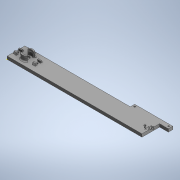
# Autodesk Inventor part: Arm Bottom Left
Saved by Autodesk Inventor 2020.5 (Build 245400000, 400)
## iProperties
Created: 2023-03-21
Part Number: Arm Bottom Left
Material: Generic
Document SubType Name: Modeling
Designer: Wes
Density: 1 g/cm^3
Appearance: Default
Author: Wes
Autodesk Inventor part; units mm, degrees
ref_plane "YZ Plane" through (0, 0, 0) normal (1, 0, 0) x (0, 1, 0)
ref_plane "XZ Plane" through (0, 0, 0) normal (0, 1, 0) x (-1, 0, 0)
ref_plane "XY Plane" through (0, 0, 0) normal (0, 0, 1) x (1, 0, 0)
sketch "Base" plane through (0, 0, 0) normal (0, 0, 1) x (1, 0, 0)
  line L0 (0, 0) -> (-30, 0)
  line L1 (-30, 0) -> (-30, 230)
  line L2 (-30, 230) -> (0, 230)
  line L3 (0, 230) -> (0, 0)
  dimension "d0" = 30
  dimension "d1" = 230
  constraints: 8 end point, 2 parallel, 1 horizontal, 1 perpendicular
  measures "d0" distance of L1.end L2.end
  measures "d1" distance of L0.end L1.end
sketch "Base outline for Extrusion1" plane through (0, 0, 0) normal (0, 0, 1) x (1, 0, 0)
  line L0 (0, 0) -> (0, 230)
  line L1 (-30, 0) -> (0, 0)
  line L2 (-30, 230) -> (-30, 0)
  line L3 (0, 230) -> (-30, 230)
extrude "Extrusion1" add sketch "Base outline for Extrusion1" along normal blind 5
sketch "Axle Screw Countersink" plane through (0, 0, 5) normal (0, 0, 1) x (1, 0, 0)
  line L0 (-15, 0) -> (-15, 20) construction
  circle A0 centre (-15, 20) radius 3.15
  dimension "d4" = 20
  dimension "d58" = 6.3
  constraints: 2 end point, 1 centre point, 1 coincident, 1 vertical
  measures "d4" distance of L0.start L0.end
  measures "d58" diameter of A0
sketch "Axle Screw Countersink outline for Extrusion2" plane through (0, 0, 5) normal (0, 0, 1) x (1, 0, 0)
  circle A0 centre (-15, 20) radius 3.15
extrude "Extrusion2" cut sketch "Axle Screw Countersink outline for Extrusion2" against normal blind 1.2
sketch "Motor Arm Center Fitting" plane through (0, 0, 5) normal (0, 0, 1) x (1, 0, 0)
  line L0 (-19.392963, 15.95) -> (-19.392963, 24.05) construction
  arc A0 (-19.392963, 24.05) -> (-19.392963, 15.95) centre (-15, 20) ccw
  line L1 (-19.392963, 15.95) -> (-21.231023, 14.255439)
  line L2 (-19.392963, 24.05) -> (-21.231023, 25.744561)
  line L3 (-15, 8.350441) -> (-15, 30.698869) construction
  arc A1 (-21.231023, 25.744561) -> (-21.231023, 14.255439) centre (-15, 20) ccw
  line L4 (-10.607037, 15.95) -> (-10.607037, 24.05) construction
  line L5 (-10.607037, 15.95) -> (-19.392963, 15.95) construction
  arc A2 (-10.607037, 15.95) -> (-10.607037, 24.05) centre (-15, 20) ccw
  line L6 (-10.607037, 15.95) -> (-8.768977, 14.255439)
  line L7 (-10.607037, 24.05) -> (-8.768977, 25.744561)
  arc A3 (-8.768977, 14.255439) -> (-8.768977, 25.744561) centre (-15, 20) ccw
  circle A4 centre (-15, 20) radius 5.975 construction
  point P0 (0, 0)
  point P1 (-15, 20)
  dimension "d18" = 11.95
  dimension "d19" = 8.1
  dimension "d20" = 8.1
  dimension "d21" = 2.5
  dimension "d22" = 2.5
  constraints: 16 end point, 12 point on circle, 5 centre point, 2 line through centre, 2 symmetric about line, 2 vertical, 1 concentric, 1 perpendicular, 2 other
  measures "d18" diameter of A4
  measures "d19" distance of L5.start L4.end
  measures "d20" distance of L5.end L0.end
  measures "d21" distance of L5.end L1.end
  measures "d22" distance of L0.end L2.end
sketch "Motor Arm Center Fitting outline for Extrusion3" plane through (0, 0, 5) normal (0, 0, 1) x (1, 0, 0)
  arc A0 (-10.607037, 24.05) -> (-10.607037, 15.95) centre (-15, 20) cw
  line L0 (-8.768977, 25.744561) -> (-10.607037, 24.05)
  arc A1 (-8.768977, 14.255439) -> (-8.768977, 25.744561) centre (-15, 20) ccw
  line L1 (-10.607037, 15.95) -> (-8.768977, 14.255439)
  arc A2 (-21.231023, 25.744561) -> (-21.231023, 14.255439) centre (-15, 20) ccw
  line L2 (-19.392963, 24.05) -> (-21.231023, 25.744561)
  arc A3 (-19.392963, 15.95) -> (-19.392963, 24.05) centre (-15, 20) cw
  line L3 (-21.231023, 14.255439) -> (-19.392963, 15.95)
extrude "Extrusion3" add sketch "Motor Arm Center Fitting outline for Extrusion3" along normal blind 5
sketch "Motor Rotation Support" plane through (0, 0, 10) normal (0, 0, 1) x (1, 0, 0)
  line L0 (-20.975, 20) -> (-21.775, 20) construction
  circle A0 centre (-15, 20) radius 6.775 construction
  arc A1 (-19.981142, 24.592259) -> (-19.981142, 15.407741) centre (-15, 20) ccw
  line L1 (-21.775, 20) -> (-23.775, 20) construction
  circle A2 centre (-15, 20) radius 8.775 construction
  arc A3 (-21.45159, 25.947908) -> (-21.45159, 14.052092) centre (-15, 20) ccw
  line L2 (-21.45159, 14.052092) -> (-19.981142, 15.407741)
  line L3 (-19.981142, 24.592259) -> (-21.45159, 25.947908)
  line L4 (-15, 8.529475) -> (-15, 32.047921) construction
  line L5 (-8.54841, 14.052092) -> (-10.018858, 15.407741)
  arc A4 (-8.54841, 14.052092) -> (-8.54841, 25.947908) centre (-15, 20) ccw
  arc A5 (-10.018858, 15.407741) -> (-10.018858, 24.592259) centre (-15, 20) ccw
  line L6 (-10.018858, 24.592259) -> (-8.54841, 25.947908)
  point P0 (0, 0)
  point P1 (-21.231023, 14.255439)
  point P2 (-21.231023, 25.744561)
  dimension "d25" = 0.8
  dimension "d26" = 2
  constraints: 16 point on circle, 14 end point, 6 centre point, 4 symmetric about line, 2 coincident, 2 horizontal, 1 concentric, 1 vertical, 2 other
  measures "d25" distance of L0.start L0.end
  measures "d26" distance of L0.end L1.end
sketch "Motor Rotation Support outline for Extrusion4" plane through (0, 0, 10) normal (0, 0, 1) x (1, 0, 0)
  arc A0 (-8.54841, 14.052092) -> (-8.54841, 25.947908) centre (-15, 20) ccw
  line L0 (-10.018858, 15.407741) -> (-8.54841, 14.052092)
  arc A1 (-10.018858, 24.592259) -> (-10.018858, 15.407741) centre (-15, 20) cw
  line L1 (-8.54841, 25.947908) -> (-10.018858, 24.592259)
  arc A2 (-21.45159, 25.947908) -> (-21.45159, 14.052092) centre (-15, 20) ccw
  line L2 (-19.981142, 24.592259) -> (-21.45159, 25.947908)
  arc A3 (-19.981142, 15.407741) -> (-19.981142, 24.592259) centre (-15, 20) cw
  line L3 (-21.45159, 14.052092) -> (-19.981142, 15.407741)
extrude "Extrusion4" add sketch "Motor Rotation Support outline for Extrusion4" along normal blind 3.35
sketch "Motor Arm Screw Holes" plane through (0, 0, 5) normal (0, 0, 1) x (1, 0, 0)
  line L0 (-15, 20) -> (-15, 37.1) construction
  line L1 (-15, 20) -> (-15, 2.9) construction
  line L2 (-15, 20) -> (-15, 4.2) construction
  line L3 (-15, 20) -> (-15, 35.8) construction
  line L4 (-15, 4.2) -> (-15, 2.9) construction
  line L5 (-15, 35.8) -> (-15, 37.1) construction
  circle A0 centre (-15, 36.45) radius 1.175
  circle A1 centre (-15, 3.55) radius 1.175
  point P0 (0, 0)
  dimension "d59" = 34.2
  dimension "d60" = 31.6
  dimension "d61" = 2.35
  dimension "d62" = 2.35
  constraints: 12 end point, 3 vertical, 2 centre point, 2 midpoint, 2 point on line, 1 coincident, 1 collinear
  measures "d59" distance of L0.end L1.end
  measures "d60" distance of L3.end L2.end
  measures "d61" diameter of A0
  measures "d62" diameter of A1
sketch "Motor Arm Screw Holes outline for Extrusion5" plane through (0, 0, 5) normal (0, 0, 1) x (1, 0, 0)
  circle A0 centre (-15, 36.45) radius 1.175
  circle A1 centre (-15, 3.55) radius 1.175
extrude "Extrusion5" cut sketch "Motor Arm Screw Holes outline for Extrusion5" against normal through all
sketch "Motor Arm Support" plane through (0, 0, 5) normal (0, 0, 1) x (1, 0, 0)
  line L0 (-15, 2.375) -> (-15, 6.875) construction
  line L1 (-15, 6.875) -> (-11.875, 6.875) construction
  line L2 (-15, 6.875) -> (-18.125, 6.875) construction
  line L3 (-21.064431, 20.215447) -> (-9.114431, 20.215447) construction
  line L4 (-15, 3.55) -> (-12.2, 3.55) construction
  line L5 (-15, 3.55) -> (-12.2, 3.55) construction
  line L6 (-15, 3.55) -> (-17.8, 3.55) construction
  line L7 (-15, 3.55) -> (-12.2, 3.55) construction
  line L8 (-18.125, 6.875) -> (-17.8, 3.55)
  line L9 (-17.8, 3.55) -> (-19.790514, 3.355438)
  line L10 (-19.790514, 3.355438) -> (-20.115514, 6.680438)
  line L11 (-20.115514, 6.680438) -> (-18.125, 6.875)
  line L12 (-11.875, 6.875) -> (-12.2, 3.55)
  line L13 (-12.2, 3.55) -> (-10.209486, 3.355438)
  line L14 (-9.884486, 6.680438) -> (-11.875, 6.875)
  line L15 (-10.209486, 3.355438) -> (-9.884486, 6.680438)
  line L16 (-17.8, 3.55) -> (-17.605438, 1.559486)
  line L17 (-17.605438, 1.559486) -> (-19.595952, 1.364925)
  line L18 (-19.595952, 1.364925) -> (-19.790514, 3.355438)
  line L19 (-12.2, 3.55) -> (-12.394562, 1.559486)
  line L20 (-12.394562, 1.559486) -> (-10.404048, 1.364925)
  line L21 (-10.404048, 1.364925) -> (-10.209486, 3.355438)
  line L22 (-17.8, 36.880894) -> (-19.790514, 37.075456)
  line L23 (-17.8, 36.880894) -> (-17.605438, 38.871408)
  line L24 (-17.605438, 38.871408) -> (-19.595952, 39.06597)
  line L25 (-19.595952, 39.06597) -> (-19.790514, 37.075456)
  line L26 (-18.125, 33.555894) -> (-17.8, 36.880894)
  line L27 (-19.790514, 37.075456) -> (-20.115514, 33.750456)
  line L28 (-20.115514, 33.750456) -> (-18.125, 33.555894)
  line L29 (-11.875, 33.555894) -> (-12.2, 36.880894)
  line L30 (-12.394562, 38.871408) -> (-10.404048, 39.06597)
  line L31 (-12.2, 36.880894) -> (-10.209486, 37.075456)
  line L32 (-10.404048, 39.06597) -> (-10.209486, 37.075456)
  line L33 (-10.209486, 37.075456) -> (-9.884486, 33.750456)
  line L34 (-9.884486, 33.750456) -> (-11.875, 33.555894)
  line L35 (-12.2, 36.880894) -> (-12.394562, 38.871408)
  point P0 (0, 0)
  dimension "d63" = 4.5
  dimension "d64" = 6.25
  dimension "d65" = 5.6
  dimension "d66" = 2
  dimension "d67" = 2
  constraints: 72 end point, 18 symmetric about line, 7 horizontal, 5 perpendicular, 2 collinear, 1 vertical
  measures "d63" distance of L0.start L1.start
  measures "d64" distance of L2.end L1.end
  measures "d65" distance of L8.end L4.end
  measures "d66" distance of L8.end L10.start
  measures "d67" distance of L8.end L17.start
sketch "Motor Arm Support outline for Extrusion6" plane through (0, 0, 5) normal (0, 0, 1) x (1, 0, 0)
  line L0 (-11.875, 6.875) -> (-12.394562, 1.559486)
  line L1 (-12.394562, 1.559486) -> (-10.404048, 1.364925)
  line L2 (-10.404048, 1.364925) -> (-9.884486, 6.680438)
  line L3 (-9.884486, 6.680438) -> (-11.875, 6.875)
  line L4 (-20.115514, 6.680438) -> (-19.595952, 1.364925)
  line L5 (-19.595952, 1.364925) -> (-17.605438, 1.559486)
  line L6 (-17.605438, 1.559486) -> (-18.125, 6.875)
  line L7 (-18.125, 6.875) -> (-20.115514, 6.680438)
  line L8 (-9.884486, 33.750456) -> (-10.404048, 39.06597)
  line L9 (-10.404048, 39.06597) -> (-12.394562, 38.871408)
  line L10 (-12.394562, 38.871408) -> (-11.875, 33.555894)
  line L11 (-11.875, 33.555894) -> (-9.884486, 33.750456)
  line L12 (-18.125, 33.555894) -> (-17.605438, 38.871408)
  line L13 (-17.605438, 38.871408) -> (-19.595952, 39.06597)
  line L14 (-19.595952, 39.06597) -> (-20.115514, 33.750456)
  line L15 (-20.115514, 33.750456) -> (-18.125, 33.555894)
extrude "Extrusion6" add sketch "Motor Arm Support outline for Extrusion6" along normal blind 3
draft "FaceDraft1" angle 28 pull direction (0, 0, 1) faces at (-10.23086, 3.136763, 6) (-10.057673, 35.522294, 6) fixed edges at (-10.144267, 4.022682, 8) (-10.144267, 36.408213, 8)
draft "FaceDraft2" angle 28 pull direction (0, 0, 1) faces at (-19.76914, 37.294132, 6) (-19.942327, 4.9086, 6) fixed edges at (-19.855733, 36.408213, 8) (-19.855733, 4.022682, 8)
fillet "Fillet1" radius 2 4 edges at (-23.475, 20, 5) (-6.525, 20, 5) (-8.225, 20, 10) (-21.775, 20, 10)
sketch "Axle Hole" plane through (0, 0, 5) normal (0, 0, 1) x (1, 0, 0)
  line L0 (0, 230) -> (-30, 230) construction
  line L1 (-15, 230) -> (-15, 220) construction
  circle A0 centre (-15, 220) radius 1.5
  point P0 (0, 0)
  dimension "d73" = 10
  dimension "d74" = 3
  constraints: 2 end point, 1 centre point, 1 coincident, 1 midpoint, 1 vertical
  measures "d73" distance of L1.start L1.end
  measures "d74" diameter of A0
sketch "Axle Hole outline for Extrusion7" plane through (0, 0, 5) normal (0, 0, 1) x (1, 0, 0)
  circle A0 centre (-15, 220) radius 1.5
extrude "Extrusion7" cut sketch "Axle Hole outline for Extrusion7" against normal through all
sketch "Motor Backplate Offset" plane through (0, 0, 0) normal (0, 0, -1) x (-1, 0, 0)
  circle A0 centre (15, 220) radius 1.5 construction
  line L0 (15, 220) -> (15, 180) construction
  line L1 (15, 220) -> (15, 240) construction
  line L2 (33.5, 240) -> (33.5, 180)
  line L3 (33.5, 180) -> (30, 180)
  line L4 (30, 180) -> (30, 240)
  line L5 (30, 240) -> (30, 245)
  line L6 (30, 245) -> (33.5, 245)
  line L7 (33.5, 245) -> (33.5, 240)
  line L8 (30, 230) -> (30, 245)
  point P0 (0, 0)
  dimension "d77" = 40
  dimension "d78" = 20
  dimension "d83" = 3.5
  dimension "d84" = 60
  dimension "d142" = 5
  constraints: 18 end point, 2 parallel, 2 vertical
  measures "d77" distance of L0.start L0.end
  measures "d78" distance of L0.start L1.end
  measures "d83" distance of L2.end L3.end
  measures "d84" distance of L0.end L1.end
  measures "d142" distance of L5.start L5.end
sketch "Motor Backplate Offset outline for Extrusion8" plane through (0, 0, 0) normal (0, 0, -1) x (-1, 0, 0)
  line L0 (30, 240) -> (30, 180)
  line L1 (30, 245) -> (30, 240)
  line L2 (33.5, 245) -> (30, 245)
  line L3 (33.5, 240) -> (33.5, 245)
  line L4 (33.5, 180) -> (33.5, 240)
  line L5 (30, 180) -> (33.5, 180)
extrude "Extrusion8" add sketch "Motor Backplate Offset outline for Extrusion8" against normal up to surface (5 mm away)
sketch "Reference" plane through (0, 0, 0) normal (0, 0, -1) x (-1, 0, 0)
  circle A0 centre (15, 220) radius 1.5 construction
  line L0 (15, 220) -> (24.935, 220) construction
  point P0 (0, 0)
  dimension "d98" = 9.935
  constraints: 2 end point, 1 horizontal
  measures "d98" distance of L0.start L0.end
sketch "Motor Backplate Offset 2" plane through (0, 0, 0) normal (0, 0, -1) x (-1, 0, 0)
  line L0 (33.5, 180) -> (33.5, 245) projected
  line L1 (33.5, 245) -> (37.5, 245)
  line L2 (37.5, 245) -> (37.5, 180)
  line L3 (37.5, 180) -> (33.5, 180)
  line L4 (33.5, 180) -> (33.5, 245)
  point P0 (0, 0)
  dimension "d144" = 4
  constraints: 8 end point, 2 parallel, 1 horizontal, 1 perpendicular
  measures "d144" distance of L2.end L3.end
sketch "Motor Backplate Offset 2 outline for Extrusion17" plane through (0, 0, 0) normal (0, 0, -1) x (-1, 0, 0)
  line L0 (33.5, 180) -> (37.5, 180)
  line L1 (33.5, 245) -> (33.5, 180)
  line L2 (37.5, 245) -> (33.5, 245)
  line L3 (37.5, 180) -> (37.5, 245)
extrude "Extrusion17" add sketch "Motor Backplate Offset 2 outline for Extrusion17" against normal up to surface (5 mm away)
sketch "Connector Screw Holes" plane through (0, 0, 0) normal (0, 0, -1) x (-1, 0, 0)
  line L0 (37.5, 180) -> (37.5, 245) construction
  line L1 (37.5, 245) -> (37.5, 241.5) construction
  line L2 (37.5, 241.5) -> (34, 241.5) construction
  line L3 (30, 180) -> (37.5, 180) construction
  line L4 (37.5, 180) -> (37.5, 183.5) construction
  line L5 (37.5, 183.5) -> (34, 183.5) construction
  circle A0 centre (34, 241.5) radius 1.275
  circle A1 centre (34, 183.5) radius 1.275
  point P0 (0, 0)
  dimension "d147" = 3.5
  dimension "d148" = 3.5
  dimension "d149" = 3.5
  dimension "d150" = 3.5
  dimension "d151" = 2.55
  dimension "d152" = 2.55
  constraints: 8 end point, 2 centre point, 2 coincident, 2 horizontal, 2 point on line
  measures "d147" distance of L0.end L1.end
  measures "d148" distance of L1.end L2.end
  measures "d149" distance of L0.start L4.end
  measures "d150" distance of L4.end L5.end
  measures "d151" diameter of A0
  measures "d152" diameter of A1
sketch "Connector Screw Holes outline for Extrusion18" plane through (0, 0, 0) normal (0, 0, -1) x (-1, 0, 0)
  circle A0 centre (34, 241.5) radius 1.275
  circle A1 centre (34, 183.5) radius 1.275
extrude "Extrusion18" cut sketch "Connector Screw Holes outline for Extrusion18" against normal up to surface (5 mm away)
body "Solid1"
